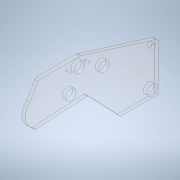
# Autodesk Inventor part: Intake-v1
Saved by Autodesk Inventor 2022 (Build 260153000, 153)
## iProperties
Created: 2022-01-09
Part Number: Intake-v1
Material: Generic
Document SubType Name: Modeling
Designer: merky
Density: 1 g/cm^3
Appearance: Polycarbonate - Clear
Mass: 272.104 g
Surface Area: 946.386 cm^2
Volume: 272.104 cm^3
Author: merky
Autodesk Inventor part; units mm, degrees
ref_plane "YZ Plane" through (0, 0, 0) normal (1, 0, 0) x (0, 1, 0)
ref_plane "XZ Plane" through (0, 0, 0) normal (0, 1, 0) x (-1, 0, 0)
ref_plane "XY Plane" through (0, 0, 0) normal (0, 0, 1) x (1, 0, 0)
sketch "Sketch1" plane through (0, 0, 0) normal (1, 0, 0) x (0, 1, 0)
  circle A0 centre (143.9084, 246.9114) radius 25.4 construction
  circle A1 centre (165.3998, 156.5759) radius 25.4 construction
  circle A2 centre (143.9084, 246.9114) radius 14.2875
  circle A3 centre (165.3998, 156.5759) radius 14.2875
  arc A4 (180.8102, 358.5299) -> (124.0141, 358.5299) centre (152.4121, 333.1299) ccw
  line L0 (127.0121, 361.528) -> (111.7556, 346.2715)
  line L1 (151.8132, 8.702) -> (48.4022, 8.702)
  line L2 (117.9037, 202.8627) -> (109.9063, 341.4154)
  arc A5 (111.7556, 346.2715) -> (109.9063, 341.4154) centre (116.2457, 341.7813) ccw
  arc A6 (116.7471, 198.8279) -> (117.9037, 202.8627) centre (111.5643, 202.4968) ccw
  arc A7 (151.8132, 8.702) -> (158.0642, 13.9355) centre (151.8132, 15.052) ccw
  circle A8 centre (44.0062, 25.4424) radius 14.2875
  line L3 (48.4022, 8.702) -> (25.3949, 8.702)
  line L4 (180.8102, 358.5299) -> (219.6983, 334.9834)
  line L5 (222.7593, 329.5515) -> (222.7593, 222.4129)
  line L6 (222.4715, 220.5229) -> (158.0642, 13.9355)
  arc A9 (222.7593, 329.5515) -> (219.6983, 334.9834) centre (216.4093, 329.5515) ccw
  arc A10 (222.4715, 220.5229) -> (222.7593, 222.4129) centre (216.4093, 222.4129) ccw
  circle A11 centre (196.3745, 222.9354) radius 14.2875
  circle A12 centre (196.3745, 197.5354) radius 2.5781
  circle A13 centre (196.3745, 248.3354) radius 2.5781
  line L7 (25.3949, 111.9383) -> (116.7471, 198.8279)
  line L8 (25.3949, 8.702) -> (25.3949, 111.9383)
  circle A14 centre (145.8462, 22.3213) radius 6.35
  point P0 (177.8121, 361.528)
  dimension "d2" = 28.575
  dimension "d3" = 28.575
  dimension "d18" = 6.35
  dimension "d19" = 28.575
  dimension "d21" = 5.1562
  dimension "d36" = 12.7
  constraints: 18 end point, 15 centre point, 14 point on circle, 8 tangent, 2 coincident, 2 vertical, 1 equal radius, 1 horizontal, 1 point on line
  measures "d2" diameter of A2
  measures "d3" diameter of A3
  measures "d18" radius of A9
  measures "d19" diameter of A11
  measures "d21" diameter of A13
  measures "d36" diameter of A14
extrude "Extrusion1" add sketch "Sketch1" along normal blind 9.525 contours L4 A9 L5 A10 L6 A7 L1 L3 L8 L7 A6 L2 A5 L0 A4
body "Solid1"
